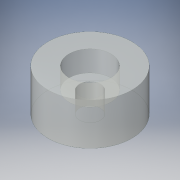
# Autodesk Inventor part: bearing base _xw
Saved by Autodesk Inventor 2016 (Build 200138000, 138)
## iProperties
Created: 2015-06-09
Part Number: bearing base _xw
Material: Generic
Document SubType Name: Modeling
Designer: 121767
Density: 1 g/cm^3
Appearance: Clear
Author: 121767
Autodesk Inventor part; units mm, degrees
ref_plane "YZ Plane" through (0, 0, 0) normal (1, 0, 0) x (0, 1, 0)
ref_plane "XZ Plane" through (0, 0, 0) normal (0, 1, 0) x (-1, 0, 0)
ref_plane "XY Plane" through (0, 0, 0) normal (0, 0, 1) x (1, 0, 0)
sketch "Sketch1" plane through (0, 0, 0) normal (1, 0, 0) x (0, 1, 0)
  line L0 (0.1359, -0.25) -> (-0.3641, -0.25)
  line L1 (-0.3641, -0.25) -> (-0.3641, -1)
  line L2 (-0.3641, -1) -> (0.6359, -1)
  line L3 (0.6359, -1) -> (0.6359, -0.5)
  line L4 (0.6359, -0.5) -> (0.1359, -0.5)
  line L5 (0.1359, -0.5) -> (0.1359, -0.25)
  line L6 (0.8485, 0) -> (-0.3641, 0)
  point P0 (0, 0)
  dimension "d0" = 1
  dimension "d2" = 2
  dimension "d3" = 1
  dimension "d4" = 0.5
  dimension "d5" = 0.5
  constraints: 14 end point, 5 perpendicular, 1 horizontal, 1 parallel, 1 point on line
  measures "d0" diameter of L4 L6
  measures "d2" diameter of L2 L6
  measures "d3" distance of L1.end L2.end
  measures "d4" distance of L3.end L4.end
  measures "d5" diameter of L0 L6
revolve "Revolution1" add sketch "Sketch1" angle 360 about axis through (0, 0.8485, 0) along (0, -1, 0)
body "Solid1"
